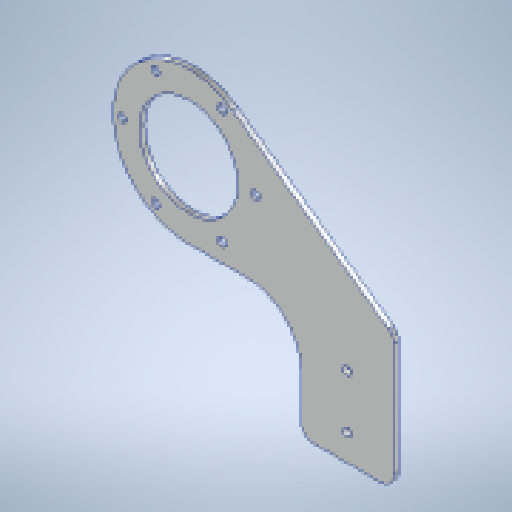
# Autodesk Inventor part: servoplate1_forR2
Saved by Autodesk Inventor 2024.3 (Build 283343010, 343A)
## iProperties
Created: 2025-05-28
Part Number: servoplate1_forR2
Material: アルミニウム 6061
Document SubType Name: Sheet Metal
Designer: kshau
Density: 2.7 g/cm^3
Appearance: アルミニウム - フラット
Mass: 14.1974 g
Surface Area: 154.294 cm^2
Volume: 14.1974 cm^3
Sheet Metal Rule: Default
Author: kshau
Autodesk Inventor part; units mm, degrees
ref_plane "YZ Plane" through (0, 0, 0) normal (1, 0, 0) x (0, 1, 0)
ref_plane "XZ Plane" through (0, 0, 0) normal (0, 1, 0) x (-1, 0, 0)
ref_plane "XY Plane" through (0, 0, 0) normal (0, 0, 1) x (1, 0, 0)
sketch "スケッチ1" plane through (0, 0, 0) normal (0, 0, 1) x (1, 0, 0)
  circle A0 centre (0, 0) radius 28.5
  line L0 (0, 0) -> (59.55, 0)
  line L1 (59.55, 0) -> (42.05, 0)
  line L2 (42.05, 0) -> (42.05, -70)
  line L3 (42.05, -70) -> (59.55, -70)
  line L4 (59.55, -70) -> (59.55, 0)
  line L5 (77.05, 0) -> (77.05, -70)
  line L6 (77.05, -70) -> (59.55, -70)
  line L7 (77.05, 0) -> (59.55, 0)
  line L8 (42.05, -70) -> (-17.7725, -22.2798)
  line L9 (77.05, -20) -> (42.05, -20)
  line L10 (77.05, -20) -> (16.5623, 23.1936)
  point P0 (42.05, 0)
  point P1 (28.5, 0)
  dimension "d0" = 57
  dimension "d1" = 59.55
  dimension "d2" = 17.5
  dimension "d3" = 70
  dimension "d31" = 50
  constraints: 22 end point, 3 horizontal, 2 parallel, 2 perpendicular, 2 point on circle, 2 point on line, 2 symmetric about line, 2 tangent, 1 centre point, 1 coincident
  measures "d0" diameter of A0
  measures "d1" distance of L0.start L0.end
  measures "d2" distance of L2.end L3.end
  measures "d3" distance of L3.end L0.end
  measures "d31" distance between parallel lines of L3 L9
extrude "押し出し1" add sketch "スケッチ1" along normal blind 2 contours A0 | L0 L2 L8 A0 | A0 L10 L0 | L0 L10 L4 L9 L2 | L2 L9 L4 L3 | L10 L9 L4 | L4 L9 L5 L6
sketch "スケッチ2" plane through (0, 0, 0) normal (0, 0, -1) x (-1, 0, 0)
  circle A0 centre (0, 0) radius 18.5
  dimension "d6" = 37
  constraints: 1 centre point, 1 coincident
  measures "d6" diameter of A0
extrude "押し出し2" cut sketch "スケッチ2" against normal blind 2
sketch "スケッチ3" plane through (0, 0, 0) normal (0, 0, -1) x (-1, 0, 0)
  arc A0 (17.7725, -22.2798) -> (-16.5623, 23.1936) centre (0, 0) ccw projected
  circle A1 centre (0, 0) radius 25
  line L0 (0, 0) -> (0, 28.5)
  line L1 (0, 0) -> (12.5, 21.6506)
  point P0 (-19.257, 34.2013)
  point P1 (12.5, 21.6506)
  point P2 (-12.5, 21.6506)
  point P3 (-25, 0)
  point P4 (-12.5, -21.6506)
  point P5 (12.5, -21.6506)
  point P6 (25, 0)
  point P7 (-39.25, 0)
  dimension "d9" = 50
  dimension "d12" = 360
  dimension "d47" = 30
  constraints: 4 end point, 3 point on circle, 1 centre point, 1 coincident, 1 point on line, 1 vertical, 7 other
  measures "d9" diameter of A1
  measures "d47" angle of L0 L1
hole "穴1" at (-12.5, 21.6506, 0) at (12.5, 21.6506, 0) at (25, 0, 0) at (12.5, -21.6506, 0) at (-12.5, -21.6506, 0) at (-25, 0, 0) direction (0, 0, 1) diameter 3.2 end through all
sketch "スケッチ4" plane through (0, 0, 0) normal (0, 0, -1) x (-1, 0, 0)
  line L0 (-77.05, -70) -> (-77.05, -20) projected
  line L1 (17.7725, -22.2798) -> (-42.05, -70) projected
  line L2 (-42.05, -70) -> (-82.05, -70)
  line L3 (-77.05, -20) -> (-42.05, -20)
  line L4 (-42.05, -20) -> (-42.05, -70)
  line L5 (-42.05, -70) -> (-77.05, -70)
  line L6 (-77.05, -70) -> (-77.05, -20)
  line L7 (-59.55, -20) -> (-59.55, -70)
  point P0 (0, 0)
  point P1 (-59.55, -40)
  point P2 (-59.55, -60)
  dimension "d32" = 20
  dimension "d33" = 20
  constraints: 12 end point, 2 midpoint, 2 parallel, 2 point on line, 1 horizontal, 1 perpendicular
  measures "d32" distance from line of L3 point (-59.55, -40)
  measures "d33" distance of point (-59.55, -40) point (-59.55, -60)
hole "穴2" at (59.55, -40, 0) at (59.55, -60, 0) direction (0, 0, 1) diameter 3.2 end through all
sketch "スケッチ5" plane through (0, 0, 0) normal (0, 0, -1) x (-1, 0, 0)
  arc A0 (17.7725, -22.2798) -> (-16.5623, 23.1936) centre (0, 0) ccw projected
  circle A1 centre (0, 0) radius 28.5
  line L0 (0, -28.5) -> (-42.05, -28.5)
  line L1 (17.7725, -22.2798) -> (-42.05, -70) projected
  line L2 (-42.05, -28.5) -> (-42.05, -70)
  point P0 (17.7725, -22.2798)
  point P1 (-2.7683, -39.25)
  point P2 (-16.5623, 23.1936)
  point P3 (17.7725, -22.2798)
  dimension "d35" = 57
  constraints: 4 end point, 2 horizontal, 1 coincident, 1 perpendicular, 3 other
extrude "押し出し3" cut sketch "スケッチ5" against normal blind 2 contours L1 L2 L0 A1
fillet "フィレット2" radius 20 1 edges at (42.05, -28.5, 1)
fillet "フィレット3" radius 5 3 edges at (42.05, -70, 1) (77.05, -70, 1) (77.05, -20, 1)
sketch "スケッチ6" plane through (0, 0, 0) normal (0, 0, -1) x (-1, 0, 0)
  circle A0 centre (12.5, 21.6506) radius 1.6 projected
  circle A1 centre (12.5, 21.6506) radius 3
  circle A2 centre (-12.5, 21.6506) radius 3
  circle A3 centre (-25, 0) radius 3
  circle A4 centre (-12.5, -21.6506) radius 3
  circle A5 centre (12.5, -21.6506) radius 3
  circle A6 centre (25, 0) radius 3
  point P0 (0, 0)
  dimension "d40" = 6
  dimension "d43" = 360
  constraints: 6 centre point, 1 coincident, 13 other
  measures "d40" diameter of A1
extrude "押し出し4" [suppressed]
equation "\"d1\" = Sside"
equation "\"BendRadius\" = Thickness"
equation "\"BendReliefWidth\" = Thickness"
equation "\"BendReliefDepth\" = 0.5 * Thickness"
equation "\"CornerReliefSize\" = 4 * Thickness"
equation "\"MinimumRemnant\" = 2 * Thickness"
equation "\"TransitionRadius\" = BendRadius"
equation "\"JacobiRadiusSize\" = BendRadius"
equation "\"GapSize\" = Thickness"
equation "\"Sside\" = 59.55"
equation "\"Thickness\" = 3.048"
